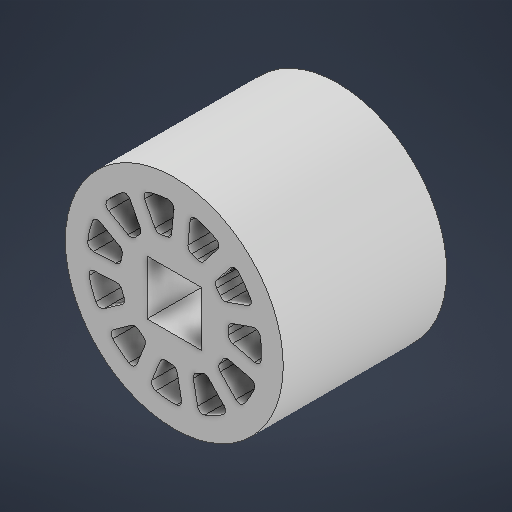
# Autodesk Inventor part: СИСЬКА
Saved by Autodesk Inventor 2025 (Build 290162000, 162)
## iProperties
Created: 2025-10-03
Part Number: СИСЬКА
Material: Типовые
Document SubType Name: Modeling
Designer: Phantom
Density: 1 g/cm^3
Appearance: По умолчанию
Author: Phantom
Autodesk Inventor part; units mm, degrees
ref_plane "YZ Plane" through (0, 0, 0) normal (1, 0, 0) x (0, 1, 0)
ref_plane "XZ Plane" through (0, 0, 0) normal (0, 1, 0) x (-1, 0, 0)
ref_plane "XY Plane" through (0, 0, 0) normal (0, 0, 1) x (1, 0, 0)
sketch "Эскиз1" plane through (0, 0, 0) normal (0, 0, 1) x (1, 0, 0)
  line L0 (-10.0069, -9.9098) -> (-10.0069, 10.0902)
  line L1 (-10.0069, 10.0902) -> (9.9931, 10.0902)
  line L2 (9.9931, 10.0902) -> (9.9931, -9.9098)
  line L3 (9.9931, -9.9098) -> (-10.0069, -9.9098)
  arc A0 (15.9207, 25.1962) -> (15.3056, 28.1887) centre (14.3486, 26.4325) ccw
  line L4 (10.8274, 18.7196) -> (15.9207, 25.1962)
  arc A1 (8.4102, 18.1432) -> (10.8274, 18.7196) centre (9.2553, 19.9559) ccw
  arc A2 (8.4102, 18.1432) -> (6.3595, 18.9642) centre (-0.0069, 0.0902) ccw
  arc A3 (5.0078, 21.0494) -> (6.3595, 18.9642) centre (6.9987, 20.8593) ccw
  line L5 (5.791, 29.2515) -> (5.0078, 21.0494)
  arc A4 (8.3012, 30.9928) -> (5.791, 29.2515) centre (7.7819, 29.0614) ccw
  arc A5 (8.3012, 30.9928) -> (-2.3164, 32.0067) centre (-0.0069, 0.0902) ccw
  arc A6 (-0.1811, 29.8218) -> (-2.3164, 32.0067) centre (-2.1721, 30.0119) ccw
  line L6 (-0.9643, 21.6197) -> (-0.1811, 29.8218)
  arc A7 (-2.6862, 19.828) -> (-0.9643, 21.6197) centre (-2.9553, 21.8098) ccw
  arc A8 (-2.6862, 19.828) -> (-4.8552, 19.4099) centre (-0.0069, 0.0902) ccw
  arc A9 (-7.1197, 20.4333) -> (-4.8552, 19.4099) centre (-5.342, 21.3498) ccw
  line L7 (-10.8952, 27.7568) -> (-7.1197, 20.4333)
  arc A10 (-9.7249, 30.5788) -> (-10.8952, 27.7568) centre (-9.1176, 28.6733) ccw
  arc A11 (-9.7249, 30.5788) -> (-19.2052, 25.6914) centre (-0.0069, 0.0902) ccw
  arc A12 (-16.2276, 25.0078) -> (-19.2052, 25.6914) centre (-18.0053, 24.0914) ccw
  line L8 (-12.4521, 17.6843) -> (-16.2276, 25.0078)
  arc A13 (-12.932, 15.2461) -> (-12.4521, 17.6843) centre (-14.2297, 16.7678) ccw
  arc A14 (-12.932, 15.2461) -> (-14.5306, 13.7218) centre (-0.0069, 0.0902) ccw
  arc A15 (-16.9889, 13.3584) -> (-14.5306, 13.7218) centre (-15.9889, 15.0905) ccw
  line L9 (-24.1245, 17.4781) -> (-16.9889, 13.3584)
  arc A16 (-24.6657, 20.4849) -> (-24.1245, 17.4781) centre (-23.1245, 19.2102) ccw
  arc A17 (-24.6657, 20.4849) -> (-29.9986, 11.2479) centre (-0.0069, 0.0902) ccw
  arc A18 (-27.1241, 12.2826) -> (-29.9986, 11.2479) centre (-28.1241, 10.5506) ccw
  line L10 (-19.9885, 8.1629) -> (-27.1241, 12.2826)
  arc A19 (-19.0741, 5.8523) -> (-19.9885, 8.1629) centre (-20.9885, 6.4309) ccw
  arc A20 (-19.0741, 5.8523) -> (-19.5948, 3.7057) centre (-0.0069, 0.0902) ccw
  arc A21 (-21.4664, 2.0709) -> (-19.5948, 3.7057) centre (-21.5616, 4.0687) ccw
  line L11 (-29.6965, 1.6789) -> (-21.4664, 2.0709)
  arc A22 (-31.7774, 3.9157) -> (-29.6965, 1.6789) centre (-29.7917, 3.6766) ccw
  arc A23 (-31.7774, 3.9157) -> (-31.2699, -6.7381) centre (-0.0069, 0.0902) ccw
  arc A24 (-29.4111, -4.3136) -> (-31.2699, -6.7381) centre (-29.3159, -6.3113) ccw
  line L12 (-21.181, -3.9215) -> (-29.4111, -4.3136)
  arc A25 (-19.1625, -5.3709) -> (-21.181, -3.9215) centre (-21.0858, -5.9193) ccw
  arc A26 (-19.1625, -5.3709) -> (-18.44, -7.4583) centre (-0.0069, 0.0902) ccw
  arc A27 (-19.1307, -9.8454) -> (-18.44, -7.4583) centre (-20.2908, -8.2163) ccw
  line L13 (-25.8424, -14.6248) -> (-19.1307, -9.8454)
  arc A28 (-28.8022, -13.868) -> (-25.8424, -14.6248) centre (-27.0025, -12.9956) ccw
  arc A29 (-28.8022, -13.868) -> (-22.6154, -22.5562) centre (-0.0069, 0.0902) ccw
  arc A30 (-22.3624, -19.5116) -> (-22.6154, -22.5562) centre (-21.2023, -21.1408) ccw
  line L14 (-15.6508, -14.7323) -> (-22.3624, -19.5116)
  arc A31 (-13.1691, -14.8603) -> (-15.6508, -14.7323) centre (-14.4907, -16.3614) ccw
  arc A32 (-13.1691, -14.8603) -> (-11.4328, -16.2257) centre (-0.0069, 0.0902) ccw
  arc A33 (-10.7233, -18.6073) -> (-11.4328, -16.2257) centre (-12.58, -17.864) ccw
  line L15 (-13.7856, -26.2565) -> (-10.7233, -18.6073)
  arc A34 (-16.6847, -27.2201) -> (-13.7856, -26.2565) centre (-15.6423, -25.5132) ccw
  arc A35 (-16.6847, -27.2201) -> (-6.7828, -31.1842) centre (-0.0069, 0.0902) ccw
  arc A36 (-8.2161, -28.4862) -> (-6.7828, -31.1842) centre (-6.3593, -29.2296) ccw
  line L16 (-5.1538, -20.837) -> (-8.2161, -28.4862)
  arc A37 (-2.9968, -19.603) -> (-5.1538, -20.837) centre (-3.297, -21.5803) ccw
  arc A38 (-2.9968, -19.603) -> (-0.7979, -19.813) centre (-0.0069, 0.0902) ccw
  arc A39 (1.0865, -21.4329) -> (-0.7979, -19.813) centre (-0.8773, -21.8114) ccw
  line L17 (2.6459, -29.5234) -> (1.0865, -21.4329)
  arc A40 (0.7279, -31.9014) -> (2.6459, -29.5234) centre (0.682, -29.9019) ccw
  arc A41 (0.7279, -31.9014) -> (11.201, -29.8829) centre (-0.0069, 0.0902) ccw
  arc A42 (8.5367, -28.3881) -> (11.201, -29.8829) centre (10.5006, -28.0096) ccw
  line L18 (6.9789, -20.3054) -> (8.5367, -28.3881)
  arc A43 (8.1187, -18.1045) -> (6.9789, -20.3054) centre (8.9427, -19.9268) ccw
  arc A44 (8.1187, -18.1045) -> (10.086, -17.0832) centre (-0.3176, 0.5517) ccw
  arc A45 (12.5497, -17.4256) -> (10.086, -17.0832) centre (11.1023, -18.8058) ccw
  line L19 (18.2351, -23.3882) -> (12.5497, -17.4256)
  arc A46 (17.9072, -26.4256) -> (18.2351, -23.3882) centre (16.7876, -24.7684) ccw
  arc A47 (17.9072, -26.4256) -> (25.6265, -19.0653) centre (-0.0069, 0.0902) ccw
  arc A48 (22.5769, -19.2482) -> (25.6265, -19.0653) centre (24.0244, -17.8681) ccw
  line L20 (16.8911, -13.2851) -> (22.5769, -19.2482)
  arc A49 (16.6646, -10.8104) -> (16.8911, -13.2851) centre (18.3385, -11.9049) ccw
  arc A50 (16.6646, -10.8104) -> (17.769, -8.8975) centre (-0.0069, 0.0902) ccw
  arc A51 (20.0254, -7.8563) -> (17.769, -8.8975) centre (19.5539, -9.7999) ccw
  line L21 (28.0326, -9.7988) -> (20.0254, -7.8563)
  arc A52 (29.3989, -12.5312) -> (28.0326, -9.7988) centre (27.5611, -11.7424) ccw
  arc A53 (29.3989, -12.5312) -> (31.9135, -2.166) centre (-0.0069, 0.0902) ccw
  arc A54 (29.447, -3.9686) -> (31.9135, -2.166) centre (29.9185, -2.025) ccw
  line L22 (21.4398, -2.0261) -> (29.447, -3.9686)
  arc A55 (19.9114, -0.0667) -> (21.4398, -2.0261) centre (21.9113, -0.0825) ccw
  arc A56 (19.9114, -0.0667) -> (19.8062, 2.1397) centre (-0.0069, 0.0902) ccw
  arc A57 (21.1415, 4.2355) -> (19.8062, 2.1397) centre (21.7956, 2.3455) ccw
  line L23 (28.9278, 6.9303) -> (21.1415, 4.2355)
  arc A58 (31.5545, 5.3703) -> (28.9278, 6.9303) centre (29.5819, 5.0403) ccw
  arc A59 (31.5545, 5.3703) -> (23.2125, 22.1098) centre (-0.0069, 0.0902) ccw
  arc A60 (26.9459, 12.7815) -> (28.2217, 15.1615) centre (26.2834, 14.6686) ccw
  line L24 (19.1717, 10.0522) -> (26.9459, 12.7815)
  arc A61 (16.8229, 10.8638) -> (19.1717, 10.0522) centre (18.5092, 11.9393) ccw
  arc A62 (16.8229, 10.8638) -> (15.5337, 12.6575) centre (0.0291, 0.1528) ccw
  arc A63 (15.5129, 15.1424) -> (15.5337, 12.6575) centre (17.0905, 13.913) ccw
  line L25 (20.5775, 21.6415) -> (15.5129, 15.1424)
  arc A64 (23.2125, 22.1098) -> (20.5775, 21.6415) centre (22.155, 20.4122) ccw
  arc A65 (23.2125, 22.1098) -> (15.3056, 28.1887) centre (-0.0069, 0.0902) ccw
  arc A66 (8.4102, 18.1432) -> (6.3595, 18.9642) centre (-0.0069, 0.0902) ccw
  arc A67 (8.4102, 18.1432) -> (10.8274, 18.7196) centre (9.2553, 19.9559) ccw
  line L26 (10.8274, 18.7196) -> (15.9207, 25.1962)
  arc A68 (15.9207, 25.1962) -> (15.3056, 28.1887) centre (14.3486, 26.4325) ccw
  arc A69 (15.3056, 28.1887) -> (8.3012, 30.9928) centre (-0.0069, 0.0902) ccw
  arc A70 (8.3012, 30.9928) -> (5.791, 29.2515) centre (7.7819, 29.0614) ccw
  line L27 (5.791, 29.2515) -> (5.0078, 21.0494)
  arc A71 (5.0078, 21.0494) -> (6.3595, 18.9642) centre (6.9987, 20.8593) ccw
  line L28 (-0.9643, 21.6197) -> (-0.1811, 29.8218)
  arc A72 (-0.1811, 29.8218) -> (-2.3164, 32.0067) centre (-2.1721, 30.0119) ccw
  arc A73 (-2.3164, 32.0067) -> (-9.7249, 30.5788) centre (-0.0069, 0.0902) ccw
  arc A74 (-9.7249, 30.5788) -> (-10.8952, 27.7568) centre (-9.1176, 28.6733) ccw
  line L29 (-10.8952, 27.7568) -> (-7.1197, 20.4333)
  arc A75 (-7.1197, 20.4333) -> (-4.8552, 19.4099) centre (-5.342, 21.3498) ccw
  arc A76 (-2.6862, 19.828) -> (-4.8552, 19.4099) centre (-0.0069, 0.0902) ccw
  arc A77 (-2.6862, 19.828) -> (-0.9643, 21.6197) centre (-2.9553, 21.8098) ccw
  circle A78 centre (-18.0936, 19.251) radius 2.48
  arc A79 (-12.932, 15.2461) -> (-14.5306, 13.7218) centre (-0.0069, 0.0902) ccw
  arc A80 (-12.932, 15.2461) -> (-12.4521, 17.6843) centre (-14.2297, 16.7678) ccw
  line L30 (-12.4521, 17.6843) -> (-16.2276, 25.0078)
  arc A81 (-16.2276, 25.0078) -> (-19.2052, 25.6914) centre (-18.0053, 24.0914) ccw
  arc A82 (-19.2052, 25.6914) -> (-24.6657, 20.4849) centre (-0.0069, 0.0902) ccw
  arc A83 (-24.6657, 20.4849) -> (-24.1245, 17.4781) centre (-23.1245, 19.2102) ccw
  line L31 (-24.1245, 17.4781) -> (-16.9889, 13.3584)
  arc A84 (-16.9889, 13.3584) -> (-14.5306, 13.7218) centre (-15.9889, 15.0905) ccw
  arc A85 (-29.9986, 11.2479) -> (-31.7774, 3.9157) centre (-0.0069, 0.0902) ccw
  arc A86 (-31.7774, 3.9157) -> (-29.6965, 1.6789) centre (-29.7917, 3.6766) ccw
  line L32 (-29.6965, 1.6789) -> (-21.4664, 2.0709)
  arc A87 (-21.4664, 2.0709) -> (-19.5948, 3.7057) centre (-21.5616, 4.0687) ccw
  arc A88 (-19.0741, 5.8523) -> (-19.5948, 3.7057) centre (-0.0069, 0.0902) ccw
  arc A89 (-19.0741, 5.8523) -> (-19.9885, 8.1629) centre (-20.9885, 6.4309) ccw
  line L33 (-19.9885, 8.1629) -> (-27.1241, 12.2826)
  arc A90 (-27.1241, 12.2826) -> (-29.9986, 11.2479) centre (-28.1241, 10.5506) ccw
  arc A91 (-31.2699, -6.7381) -> (-28.8022, -13.868) centre (-0.0069, 0.0902) ccw
  arc A92 (-28.8022, -13.868) -> (-25.8424, -14.6248) centre (-27.0025, -12.9956) ccw
  line L34 (-25.8424, -14.6248) -> (-19.1307, -9.8454)
  arc A93 (-19.1307, -9.8454) -> (-18.44, -7.4583) centre (-20.2908, -8.2163) ccw
  arc A94 (-19.1625, -5.3709) -> (-18.44, -7.4583) centre (-0.0069, 0.0902) ccw
  arc A95 (-19.1625, -5.3709) -> (-21.181, -3.9215) centre (-21.0858, -5.9193) ccw
  line L35 (-21.181, -3.9215) -> (-29.4111, -4.3136)
  arc A96 (-29.4111, -4.3136) -> (-31.2699, -6.7381) centre (-29.3159, -6.3113) ccw
  arc A97 (-6.7828, -31.1842) -> (0.7279, -31.9014) centre (-0.0069, 0.0902) ccw
  arc A98 (0.7279, -31.9014) -> (2.6459, -29.5234) centre (0.682, -29.9019) ccw
  line L36 (2.6459, -29.5234) -> (1.0865, -21.4329)
  arc A99 (1.0865, -21.4329) -> (-0.7979, -19.813) centre (-0.8773, -21.8114) ccw
  arc A100 (-2.9968, -19.603) -> (-0.7979, -19.813) centre (-0.0069, 0.0902) ccw
  arc A101 (-2.9968, -19.603) -> (-5.1538, -20.837) centre (-3.297, -21.5803) ccw
  line L37 (-5.1538, -20.837) -> (-8.2161, -28.4862)
  arc A102 (-8.2161, -28.4862) -> (-6.7828, -31.1842) centre (-6.3593, -29.2296) ccw
  arc A103 (11.201, -29.8829) -> (17.9072, -26.4256) centre (-0.0069, 0.0902) ccw
  arc A104 (17.9072, -26.4256) -> (18.2351, -23.3882) centre (16.7876, -24.7684) ccw
  line L38 (18.2351, -23.3882) -> (12.5497, -17.4256)
  arc A105 (12.5497, -17.4256) -> (10.086, -17.0832) centre (11.1023, -18.8058) ccw
  arc A106 (8.1187, -18.1045) -> (10.086, -17.0832) centre (-0.3176, 0.5517) ccw
  arc A107 (8.1187, -18.1045) -> (6.9789, -20.3054) centre (8.9427, -19.9268) ccw
  line L39 (6.9789, -20.3054) -> (8.5367, -28.3881)
  arc A108 (8.5367, -28.3881) -> (11.201, -29.8829) centre (10.5006, -28.0096) ccw
  circle A109 centre (-16.3987, -20.5393) radius 2.48
  arc A110 (-22.6154, -22.5562) -> (-16.6847, -27.2201) centre (-0.0069, 0.0902) ccw
  arc A111 (-16.6847, -27.2201) -> (-13.7856, -26.2565) centre (-15.6423, -25.5132) ccw
  line L40 (-13.7856, -26.2565) -> (-10.7233, -18.6073)
  arc A112 (-10.7233, -18.6073) -> (-11.4328, -16.2257) centre (-12.58, -17.864) ccw
  arc A113 (-13.1691, -14.8603) -> (-11.4328, -16.2257) centre (-0.0069, 0.0902) ccw
  arc A114 (-13.1691, -14.8603) -> (-15.6508, -14.7323) centre (-14.4907, -16.3614) ccw
  line L41 (-15.6508, -14.7323) -> (-22.3624, -19.5116)
  arc A115 (-22.3624, -19.5116) -> (-22.6154, -22.5562) centre (-21.2023, -21.1408) ccw
  arc A116 (16.6646, -10.8104) -> (17.769, -8.8975) centre (-0.0069, 0.0902) ccw
  arc A117 (16.6646, -10.8104) -> (16.8911, -13.2851) centre (18.3385, -11.9049) ccw
  line L42 (16.8911, -13.2851) -> (22.5769, -19.2482)
  arc A118 (22.5769, -19.2482) -> (25.6265, -19.0653) centre (24.0244, -17.8681) ccw
  arc A119 (25.6265, -19.0653) -> (29.3989, -12.5312) centre (-0.0069, 0.0902) ccw
  arc A120 (29.3989, -12.5312) -> (28.0326, -9.7988) centre (27.5611, -11.7424) ccw
  line L43 (28.0326, -9.7988) -> (20.0254, -7.8563)
  arc A121 (20.0254, -7.8563) -> (17.769, -8.8975) centre (19.5539, -9.7999) ccw
  circle A122 centre (26.3182, 1.2115) radius 2.48
  line L44 (21.4398, -2.0261) -> (29.447, -3.9686)
  arc A123 (29.447, -3.9686) -> (31.9135, -2.166) centre (29.9185, -2.025) ccw
  arc A124 (31.9135, -2.166) -> (31.5545, 5.3703) centre (-0.0069, 0.0902) ccw
  arc A125 (31.5545, 5.3703) -> (28.9278, 6.9303) centre (29.5819, 5.0403) ccw
  line L45 (28.9278, 6.9303) -> (21.1415, 4.2355)
  arc A126 (21.1415, 4.2355) -> (19.8062, 2.1397) centre (21.7956, 2.3455) ccw
  arc A127 (19.9114, -0.0667) -> (19.8062, 2.1397) centre (-0.0069, 0.0902) ccw
  arc A128 (19.9114, -0.0667) -> (21.4398, -2.0261) centre (21.9113, -0.0825) ccw
  circle A129 centre (-0.0069, 0.0902) radius 40
  point P0 (0, 0)
  point P1 (-1.2221, -0.4307)
  point P2 (15.3056, 28.1887)
  point P3 (5.0078, 21.0494)
  point P4 (-2.3164, 32.0067)
  point P5 (-4.8552, 19.4099)
  point P6 (-7.1197, 20.4333)
  point P7 (-9.7249, 30.5788)
  point P8 (-16.9889, 13.3584)
  point P9 (-31.7774, 3.9157)
  point P10 (-31.2699, -6.7381)
  point P11 (-28.8022, -13.868)
  point P12 (-22.6154, -22.5562)
  point P13 (-6.7828, -31.1842)
  point P14 (0.7279, -31.9014)
  point P15 (11.201, -29.8829)
  point P16 (17.9072, -26.4256)
  point P17 (21.4398, -2.0261)
  dimension "d0" = 80
  constraints: 253 point on circle, 130 centre point, 92 end point, 1 coincident
  measures "d0" diameter of A129
extrude "Выдавливание1" add sketch "Эскиз1" along normal blind 60 contours A0 A65 A64 L25 A63 A62 A61 L24 A60 A59 A58 L23 A57 A56 A55 L22 A54 A53 A52 L21 A51 A50 A49 L20 A48 A47 A46 L19 A45 A44 A43 L18 A42 A41 A40 L17 A39 A38 A37 L16 A36 A35 A34 L15 A33 A32 A31 L14 A30 A29 A28 L13 A27 A26 A25 L12 A24 A23 A22 L11 A21 A20 A19 L10 A18 A17 A16 L9 A15 A14 A13 L8 A12 A11 A10 L7 A9 A8 A7 L6 A6 A5 A4 L5 A3 A2 A1 L4 | A129
